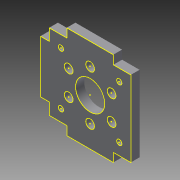
# Autodesk Inventor part: motor mount
Saved by Autodesk Inventor 2015 (Build 190159000, 159)
## iProperties
Created: 2015-10-16
Part Number: motor mount
Material: Polycarbonate, Clear
Document SubType Name: Modeling
Designer: Brian
Density: 1.2 g/cm^3
Appearance: Default
Mass: 2.62359 g
Surface Area: 22.1254 cm^2
Volume: 2.18632 cm^3
Author: Brian
Autodesk Inventor part; units mm, degrees
ref_plane "YZ Plane" through (0, 0, 0) normal (1, 0, 0) x (0, 1, 0)
ref_plane "XZ Plane" through (0, 0, 0) normal (0, 1, 0) x (-1, 0, 0)
ref_plane "XY Plane" through (0, 0, 0) normal (0, 0, 1) x (1, 0, 0)
sketch "Sketch1" plane through (0, 0, 0) normal (0, 1, 0) x (-1, 0, 0)
  circle A0 centre (0, 0) radius 11 construction
  circle A1 centre (0, 0) radius 8.5 construction
  circle A2 centre (0, -8.5) radius 1.5
  circle A3 centre (7.3612, -4.25) radius 1.5
  circle A4 centre (7.3612, 4.25) radius 1.5
  circle A5 centre (0, 8.5) radius 1.5
  circle A6 centre (-7.3612, 4.25) radius 1.5
  circle A7 centre (-7.3612, -4.25) radius 1.5
  circle A8 centre (0, 0) radius 5
  line L0 (14, 16) -> (-14, 16) construction
  line L1 (-14, 16) -> (-14, -16) construction
  line L2 (-14, -16) -> (14, -16) construction
  line L3 (14, -16) -> (14, 16) construction
  line L4 (11, 16) -> (11, -16) construction
  line L5 (14, 13) -> (-14, 13) construction
  line L6 (-11, 16) -> (-11, -16) construction
  line L7 (14, -13) -> (-14, -13) construction
  line L8 (8, 16) -> (-8, 16)
  line L9 (-8, 16) -> (-8, 13)
  line L10 (-8, 13) -> (-14, 13)
  line L11 (-14, 13) -> (-14, -13)
  line L12 (-14, -13) -> (-8, -13)
  line L13 (-8, -13) -> (-8, -16)
  line L14 (-8, -16) -> (8, -16)
  line L15 (8, -16) -> (8, -13)
  line L16 (8, -13) -> (14, -13)
  line L17 (14, 13) -> (8, 13)
  line L18 (8, 13) -> (8, 16)
  circle A9 centre (0, 0) radius 25 construction
  line L19 (14, 13) -> (14, 9)
  line L20 (14, 9) -> (17, 9)
  line L21 (17, 9) -> (17, -9)
  line L22 (17, -9) -> (14, -9)
  line L23 (14, -9) -> (14, -13)
  circle A10 centre (10, 9) radius 0.9
  circle A11 centre (-10, 9) radius 0.9
  circle A12 centre (10, -9) radius 0.9
  circle A13 centre (-10, -9) radius 0.9
  point P0 (0, -16)
  point P1 (14, 0)
  point P2 (0, 16)
  point P3 (17, 0)
  dimension "d1" = 17
  dimension "d0" = 22
  dimension "d3" = 3
  dimension "d6" = 360
  dimension "d8" = 10
  dimension "d9" = 28
  dimension "d10" = 32
  dimension "d11" = 3
  dimension "d12" = 3
  dimension "d13" = 3
  dimension "d14" = 3
  dimension "d16" = 50
  dimension "d19" = 6
  dimension "d20" = 3
  dimension "d21" = 4
  dimension "d22" = 1.8
  dimension "d23" = 4
  dimension "d24" = 4
  dimension "d25" = 1.8
  dimension "d26" = 4
  dimension "d27" = 1.8
  dimension "d28" = 4
  dimension "d29" = 1.8
  constraints: 48 end point, 20 point on line, 13 centre point, 11 perpendicular, 6 vertical alignment, 4 coincident, 4 collinear, 4 horizontal alignment, 4 midpoint, 2 horizontal, 2 parallel, 15 other
  measures "d0" diameter of A0
  measures "d3" diameter of A2
  measures "d8" diameter of A8
  measures "d9" distance of L1.end L2.end
  measures "d10" distance of L0.end L1.end
  measures "d11" distance between parallel lines of L3 L4
  measures "d12" distance between parallel lines of L0 L5
  measures "d13" distance between parallel lines of L2 L7
  measures "d14" distance between parallel lines of L1 L6
  measures "d16" diameter of A9
  measures "d19" distance between parallel lines of L18 L3
  measures "d20" distance of L19.end L20.end
  measures "d21" distance between parallel lines of L5 L20
  measures "d22" diameter of A10
  measures "d23" distance from line of L5 A10.centre
  measures "d24" distance from line of L3 A10.centre
  measures "d25" diameter of A11
  measures "d26" distance from line of A11.centre L11
  measures "d27" diameter of A12
  measures "d28" distance from line of L7 A12.centre
  measures "d29" diameter of A13
extrude "Extrusion1" add sketch "Sketch1" along normal blind 3
sketch "Sketch3" plane through (0, 0, 0) normal (0, -1, 0) x (1, 0, 0)
  circle A0 centre (0, 0) radius 5 projected
  circle A1 centre (10, -9) radius 0.9 projected
  circle A2 centre (-10, -9) radius 0.9 projected
  circle A3 centre (10, 9) radius 0.9 projected
  circle A4 centre (-10, 9) radius 0.9 projected
  circle A5 centre (7.3612, -4.25) radius 1.5 projected
  circle A6 centre (7.3612, 4.25) radius 1.5 projected
  circle A7 centre (0, 8.5) radius 1.5 projected
  circle A8 centre (-7.3612, 4.25) radius 1.5 projected
  circle A9 centre (-7.3612, -4.25) radius 1.5 projected
  circle A10 centre (0, -8.5) radius 1.5 projected
  line L0 (-14, 13) -> (-8, 13) projected
  line L1 (-14, 9) -> (-14, 13) projected
  line L2 (-17, 9) -> (-14, 9) projected
  line L3 (-17, -9) -> (-17, 9) projected
  line L4 (-14, -9) -> (-17, -9) projected
  line L5 (-14, -13) -> (-14, -9) projected
  line L6 (-8, -13) -> (-14, -13) projected
  line L7 (-8, -16) -> (-8, -13) projected
  line L8 (8, -16) -> (-8, -16) projected
  line L9 (8, -13) -> (8, -16) projected
  line L10 (14, -13) -> (8, -13) projected
  line L11 (14, 13) -> (14, -13) projected
  line L12 (8, 13) -> (14, 13) projected
  line L13 (8, 16) -> (8, 13) projected
  line L14 (-8, 16) -> (8, 16) projected
  line L15 (-8, 13) -> (-8, 16) projected
equation "\"d12\" = d11"
equation "\"d13\" = d11"
equation "\"d14\" = d11"
equation "\"d20\" = d11"
equation "\"d24\" = d23"
equation "\"d25\" = d22"
equation "\"d26\" = d24"
equation "\"d27\" = d22"
equation "\"d28\" = d23"
equation "\"d29\" = d22"
body "Solid1"
